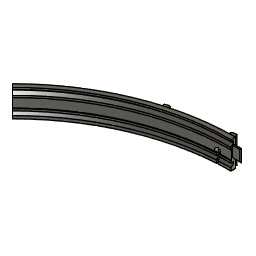
Model_LowerSegment (Autodesk Fusion 360 design; units mm, degrees)
Autodesk Fusion 360 part; units mm, degrees
sketch "Sketch1" plane through (0, 0, 0) normal (0, 0, 1) x (1, 0, 0)
  circle A0 centre (0, 0) radius 246.5
  circle A1 centre (0, 0) radius 241.5
  line L0 (0, 350) -> (0, -350)
  line L1 (-247.4874, 247.4874) -> (247.4874, -247.4874)
  line L2 (-350, 0) -> (350, 0)
  line L3 (-247.4874, -247.4874) -> (247.4874, 247.4874)
  line L4 (0, 350) -> (0, -350)
  dimension "d2" = 5
  dimension "d3" = 350
  dimension "d4" = 350
  dimension "d5" = 45
  dimension "d6" = 45
  dimension "d7" = 45
  dimension "d8" = 45
  dimension "d50" = 483
  constraint coincident A0.centre A1.centre
  constraint concentric A0 A1
  constraint vertical L0
  constraint vertical L4
  measures "d2" distance of A0 A1
  measures "d3" distance of A0.centre L0.start
  measures "d4" distance of A0.centre L0.end
  measures "d5" angle of L0 L1
  measures "d6" angle of L1 L2
  measures "d7" angle of L2 L3
  measures "d8" angle of L3 L4
  measures "d50" diameter of A1
extrude "Extrude1" add sketch "Sketch1" along normal blind 30 contours A0 A1 L0 L1 L4 picked at (-165.0426, 180.2099)
sketch "Sketch2" plane through (0, 0, 0) normal (1, 0, 0) x (0, 1, 0)
  line L0 (241.5, 0) -> (246.5, 0)
  line L1 (246.5, 0) -> (246.5, 30)
  line L2 (246.5, 30) -> (241.5, 30)
  line L3 (241.5, 30) -> (241.5, 0)
  line L4 (241.5, 28) -> (244.5, 28)
  line L5 (244.5, 28) -> (244.5, 25.5)
  line L6 (244.5, 6.1) -> (244.5, 7.6)
  line L7 (244.5, 7.6) -> (241.5, 7.6)
  line L8 (241.5, 20.3) -> (242.3, 20.3)
  line L9 (242.3, 20.3) -> (242.3, 9.8)
  line L10 (242.3, 9.8) -> (241.5, 9.8)
  line L11 (241.5, 9.8) -> (241.5, 20.3)
  line L12 (244.5, 6.1) -> (241.5, 3.1)
  line L13 (244.5, 6.1) -> (267.2426, 6.1) construction
  line L14 (244.5, 25.5) -> (241.5, 22.5)
  line L15 (244.5, 25.5) -> (267.2426, 25.5) construction
  line L16 (241.5, 28) -> (241.5, 22.5)
  line L17 (241.5, 7.6) -> (241.5, 3.1)
  dimension "d11" = 2
  dimension "d12" = 2
  dimension "d13" = 2.5
  dimension "d15" = 2
  dimension "d16" = 1.5
  dimension "d17" = 10.5
  dimension "d18" = 0.8
  dimension "d20" = 2.2
  dimension "d23" = 3.1
  dimension "d25" = 2.2
  dimension "d109" = 45
  dimension "d110" = 45
  constraint horizontal L4
  constraint vertical L5
  constraint coincident L3 L4.start
  constraint vertical L6
  constraint horizontal L7
  constraint horizontal L8
  constraint vertical L9
  constraint horizontal L10
  constraint vertical L11
  constraint coincident L3 L8.start
  constraint horizontal L13
  constraint coincident L3 L12.end
  constraint horizontal L15
  constraint coincident L3 L14.end
  measures "d11" distance of L2 L4
  measures "d12" distance of L1 L5
  measures "d13" distance of L4.end L5.end
  measures "d15" distance of L1 L6
  measures "d16" distance of L6.start L6.end
  measures "d17" distance of L8.end L9.end
  measures "d18" distance of L9 L11
  measures "d20" distance of L7 L10
  measures "d23" distance of L0.start L12.end
  measures "d25" distance of L8.start L14.end
  measures "d109" angle of L14 L16
  measures "d110" angle of L12 L17
revolve "Revolve1" cut sketch "Sketch2" angle 360 about axis through (0, 0, 1.75) along (0, 0, 1) contours L3 L6 L7 L12 L17 | L3 L8 L9 L10 L11 | L3 L4 L5 L14 L16
sketch "Sketch3" plane through (0, 0, 0) normal (1, 0, 0) x (0, 1, 0)
  line L0 (241.5, 7.6) -> (244.5, 7.6)
  line L1 (244.5, 7.6) -> (244.5, 6.1)
  line L2 (244.5, 6.1) -> (241.5, 3.1)
  line L3 (241.5, 3.1) -> (241.5, 0)
  line L4 (241.5, 0) -> (246.5, 0)
  line L5 (246.5, 0) -> (246.5, 30)
  line L6 (246.5, 30) -> (241.5, 30)
  line L7 (241.5, 30) -> (241.5, 28)
  line L8 (241.5, 28) -> (244.5, 28)
  line L9 (244.5, 28) -> (244.5, 25.5)
  line L10 (244.5, 25.5) -> (241.5, 22.5)
  line L11 (241.5, 22.5) -> (241.5, 20.3)
  line L12 (241.5, 20.3) -> (242.3, 20.3)
  line L13 (242.3, 20.3) -> (242.3, 9.8)
  line L14 (242.3, 9.8) -> (241.5, 9.8)
  line L15 (241.5, 9.8) -> (241.5, 7.6)
  line L16 (245.2, 23.75) -> (243.4, 23.75)
  line L17 (245.2, 23.75) -> (245.2, 10.15)
  line L18 (245.2, 10.15) -> (243.4, 11.95)
  line L19 (245.2, 10.15) -> (249.7456, 10.15) construction
  line L20 (243.4, 23.75) -> (243.4, 11.95)
  line L21 (245.3, 23.85) -> (245.3, 9.85)
  line L22 (245.3, 9.85) -> (243.3, 11.85)
  line L23 (243.3, 11.85) -> (243.3, 23.85)
  line L24 (245.3, 23.85) -> (243.3, 23.85)
  dimension "d30" = 6.25
  dimension "d46" = 1.8
  dimension "d47" = 1.3
  dimension "d56" = 11.8
  dimension "d57" = 6.15
  dimension "d58" = 1.2
  dimension "d59" = 1.8
  dimension "d61" = 11.85
  dimension "d62" = 45
  dimension "d63" = 135
  constraint horizontal L16
  constraint perpendicular L16 L17
  constraint horizontal L19
  constraint perpendicular L16 L20
  constraint perpendicular L19 L21
  constraint perpendicular L23 L24
  measures "d30" distance of L6 L16
  measures "d46" distance of L17 L20
  measures "d47" distance of L5 L17
  measures "d56" distance of L16.end L18.end
  measures "d57" distance of L6 L24
  measures "d58" distance of L5 L21
  measures "d59" distance of L11 L23
  measures "d61" distance of L4 L22.end
  measures "d62" angle of L17 L18
  measures "d63" angle of L21 L22
revolve "Revolve2" add sketch "Sketch3" angle 1.9 about axis through (0, 0, 1.75) along (0, 0, -1) contours L16 L17 L18 L20
sketch "Sketch4" plane through (0, 0, 0) normal (-0.707107, -0.707107, 0) x (0.707107, -0.707107, 0)
  line L0 (-244.5, 7.6) -> (-241.5, 7.6)
  line L1 (-241.5, 7.6) -> (-241.5, 9.8)
  line L2 (-241.5, 9.8) -> (-242.3, 9.8)
  line L3 (-242.3, 9.8) -> (-242.3, 20.3)
  line L4 (-242.3, 20.3) -> (-241.5, 20.3)
  line L5 (-241.5, 20.3) -> (-241.5, 22.5)
  line L6 (-241.5, 22.5) -> (-244.5, 25.5)
  line L7 (-244.5, 25.5) -> (-244.5, 28)
  line L8 (-244.5, 28) -> (-241.5, 28)
  line L9 (-241.5, 28) -> (-241.5, 30)
  line L10 (-241.5, 30) -> (-246.5, 30)
  line L11 (-246.5, 30) -> (-246.5, 0)
  line L12 (-246.5, 0) -> (-241.5, 0)
  line L13 (-241.5, 0) -> (-241.5, 3.1)
  line L14 (-241.5, 3.1) -> (-244.5, 6.1)
  line L15 (-244.5, 6.1) -> (-244.5, 7.6)
  line L16 (-245.3, 23.85) -> (-243.3, 23.85)
  line L17 (-245.3, 9.85) -> (-245.3, 23.85)
  line L18 (-245.3, 9.85) -> (-243.3, 11.85)
  line L19 (-245.3, 9.85) -> (-242.4716, 9.85) construction
  line L20 (-243.3, 23.85) -> (-243.3, 11.85)
  dimension "d38" = 14
  dimension "d39" = 2
  dimension "d40" = 1.2
  dimension "d42" = 6.15
  dimension "d55" = 12
  constraint horizontal L16
  constraint vertical L17
  constraint horizontal L19
  constraint perpendicular L16 L20
  measures "d38" distance of L16.start L17.start
  measures "d39" distance of L16.start L16.end
  measures "d40" distance of L11 L17
  measures "d42" distance of L10 L16
  measures "d55" distance of L16.end L18.end
revolve "Revolve3" cut sketch "Sketch4" angle 2 about axis through (0, 0, 1.75) along (0, 0, -1) contours L16 L17 L18 L20
ref_plane "WorkPlane1" through (-43.9859, 242.5438, 22.9951) normal (-0.178442, 0.98395, 0) x (0.98395, 0.178442, 0)
sketch "Sketch5" plane through (-43.9859, 242.5438, 23.1817) normal (-0.178442, 0.98395, 0) x (0.98395, 0.178442, 0)
  line L0 (42.5862, -5.8183) -> (40.5862, -5.8183)
  line L1 (40.5862, -5.8183) -> (40.5862, 23.1817)
  line L2 (40.5862, 23.1817) -> (42.5862, 23.1817)
  line L3 (42.5862, 23.1817) -> (42.5862, -5.8183)
  line L4 (-140.4016, -6.8183) -> (43.9859, -6.8183)
  line L5 (42.5862, -5.8183) -> (36.5862, -5.8183)
  line L6 (36.5862, -5.8183) -> (36.5862, -4.8183)
  line L7 (36.5862, -4.8183) -> (42.5862, -4.8183)
  line L8 (42.5862, -4.8183) -> (42.5862, -5.8183)
  line L9 (-27.9138, -5.8183) -> (-25.9138, -5.8183)
  line L10 (-25.9138, -5.8183) -> (-25.9138, 23.1817)
  line L11 (-25.9138, 23.1817) -> (-27.9138, 23.1817)
  line L12 (-27.9138, 23.1817) -> (-27.9138, -5.8183)
  line L13 (-27.9138, -5.8183) -> (-21.9138, -5.8183)
  line L14 (-21.9138, -5.8183) -> (-21.9138, -4.8183)
  line L15 (-21.9138, -4.8183) -> (-27.9138, -4.8183)
  line L16 (-27.9138, -4.8183) -> (-27.9138, -5.8183)
  circle A0 centre (28.6336, 11.6817) radius 1.25
  line L17 (-140.4016, 23.1817) -> (43.9859, 23.1817)
  line L18 (29.3798, 12.6846) -> (29.3798, 23.1817)
  line L19 (27.8798, 12.6788) -> (27.8798, 23.1817)
  dimension "d65" = 1
  dimension "d66" = 2
  dimension "d67" = 6
  dimension "d68" = 1
  dimension "d76" = 29
  dimension "d77" = 2
  dimension "d78" = 1
  dimension "d79" = 29
  dimension "d80" = 6
  dimension "d81" = 1
  dimension "d82" = 66.5
  dimension "d100" = 2.5
  dimension "d101" = 11.5
  dimension "d106" = 1.5
  constraint horizontal L0
  constraint vertical L1
  constraint horizontal L2
  constraint vertical L3
  constraint horizontal L5
  constraint vertical L6
  constraint horizontal L7
  constraint vertical L8
  constraint horizontal L9
  constraint vertical L10
  constraint horizontal L11
  constraint vertical L12
  constraint horizontal L13
  constraint vertical L14
  constraint horizontal L15
  constraint vertical L16
  constraint coincident A0 L18.start
  constraint coincident L17 L18.end
  constraint perpendicular L17 L18
  constraint coincident A0 L19.start
  constraint coincident L17 L19.end
  constraint perpendicular L17 L19
  measures "d65" distance of L0 L4
  measures "d66" distance of L1.end L2.end
  measures "d67" distance of L0.start L5.end
  measures "d68" distance of L0.start L7.end
  measures "d76" distance of L0.start L2.end
  measures "d77" distance of L9.start L9.end
  measures "d78" distance of L4 L9
  measures "d79" distance of L9.end L10.end
  measures "d80" distance of L9.start L13.end
  measures "d81" distance of L9.start L15.end
  measures "d82" distance of L1 L10
  measures "d100" diameter of A0
  measures "d101" distance of A0.centre L17
  measures "d106" distance of L18 L19
extrude "Extrude7" cut sketch "Sketch5" against normal blind 22 contours A0 | A0 L17 L18 L19
extrude "Extrude3" add sketch "Sketch5" along normal blind -5 and the other way blind -1 contours L0 L1 L3 L5 L7 L8 | L1 L5 L6 L7 | L1 L2 L3 L7 L17
sketch "Sketch6" plane through (39.9348, 7.2423, 0) normal (-0.98395, -0.178442, 0) x (0.178442, -0.98395, 0)
  line L0 (-243.1358, 0) -> (-243.1358, 28)
  line L1 (-243.1358, 28) -> (-247.5, 28)
  line L2 (-247.5, 28) -> (-247.5, 0)
  line L3 (-247.5, 0) -> (-243.1358, 0)
  line L4 (-247.5, 0) -> (-246, 0)
  line L5 (-246, 0) -> (-246, 28)
  line L6 (-246, 28) -> (-247.5, 28)
  line L7 (-247.5, 28) -> (-247.5, 0)
  dimension "d85" = 1.5
  constraint horizontal L4
  constraint vertical L5
  constraint horizontal L6
  constraint vertical L7
  constraint coincident L2.end L3.start
  measures "d85" distance of L2.end L4.end
extrude "Extrude4" add sketch "Sketch6" along normal blind 4 contours L1 L2 L3 L4 L5 L6 L7
extrude "Extrude5" add sketch "Sketch5" along normal blind -2 and the other way blind -2.7 contours L9 L10 L12 L13 L15 L16 | L10 L13 L14 L15 | L10 L11 L12 L15 L17
sketch "Sketch7" plane through (-25.4979, -4.6241, 0) normal (0.98395, 0.178442, 0) x (-0.178442, 0.98395, 0)
  line L0 (245.1341, 28) -> (245.1341, 0)
  line L1 (245.1341, 0) -> (249.2, 0)
  line L2 (249.2, 0) -> (249.2, 28)
  line L3 (249.2, 28) -> (245.1341, 28)
  line L4 (249.2, 0) -> (247.7, 0)
  line L5 (247.7, 0) -> (247.7, 28)
  line L6 (247.7, 28) -> (249.2, 28)
  line L7 (249.2, 28) -> (249.2, 0)
  constraint horizontal L4
  constraint vertical L5
  constraint horizontal L6
  constraint vertical L7
  constraint coincident L3 L5.end
  constraint coincident L1.end L2.start
extrude "Extrude6" add sketch "Sketch7" along normal blind 4 contours L1 L2 L3 L4 L5 L6 L7
fillet "Fillet3" radius 1 2 edges at (-71.9335, 240.2195, 14.5) (-66.0298, 241.2901, 14.5)
fillet "Fillet4" radius 1 2 edges at (-8.1653, 250.0563, 14.5) (-2.2616, 251.1269, 14.5)
fillet "Fillet7" radius 2 1 edges at (-14.7544, 241.8504, 12.75)
fillet "Fillet8" radius 2 1 edges at (-15.5091, 246.0116, 12.75)
